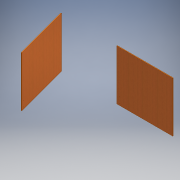
# Autodesk Inventor part: puerta
Saved by Autodesk Inventor 2016 (Build 200138000, 138)
## iProperties
Created: 2015-11-25
Part Number: puerta
Material: Generic
Document SubType Name: Modeling
Designer: Daniela
Density: 1 g/cm^3
Appearance: Glossy - Black
Author: Daniela
Autodesk Inventor part; units mm, degrees
ref_plane "YZ Plane" through (0, 0, 0) normal (1, 0, 0) x (0, 1, 0)
ref_plane "XZ Plane" through (0, 0, 0) normal (0, 1, 0) x (-1, 0, 0)
ref_plane "XY Plane" through (0, 0, 0) normal (0, 0, 1) x (1, 0, 0)
ref_plane "Plano de trabajo4" through (0, 0, 1220) normal (0, 0, 1) x (1, 0, 0)
sketch "Boceto8" plane through (0, 0, 1220) normal (0, 0, 1) x (1, 0, 0)
  line L0 (480, 0) -> (0, 0) projected
  line L1 (480, 0) -> (480, 10) projected
  line L2 (0, 10) -> (480, 10) projected
  line L3 (0, 0) -> (0, 10) projected
  line L4 (480, 10) -> (0, 10) projected
  line L5 (0, 10) -> (0, 300)
  line L6 (0, 300) -> (721.6667, 300)
  line L7 (721.6667, 300) -> (721.6667, 310)
  line L8 (721.6667, 310) -> (0, 310)
  line L9 (0, 310) -> (0, 300)
  point P0 (0, 0)
  dimension "d38" = 290
  dimension "d39" = 721.6667
  dimension "d40" = 10
  constraints: 10 end point, 2 parallel, 1 horizontal, 1 perpendicular, 1 vertical
  measures "d38" distance of L2.start L5.end
  measures "d39" distance of L8.end L7.end
  measures "d40" distance of L7.end L6.end
extrude "Extrusión8" add sketch "Boceto8" along normal blind 730 contours L9 L8 L7 L6
sketch "Boceto9" plane through (0, 300, 1220) normal (0, -1, 0) x (1, 0, 0)
  line L0 (0, 0) -> (721.6667, 0) construction
  line L1 (721.6667, 0) -> (721.6667, 730) construction
  line L2 (0, 730) -> (721.6667, 730) construction
  line L3 (0, 0) -> (0, 730) construction
  line L4 (0, 80) -> (721.6667, 80) construction
  line L5 (0, 0) -> (721.6667, 0) construction
  line L6 (36.0833, 0) -> (36.0833, 730) construction
  line L7 (0, 730) -> (721.6667, 730) construction
  circle A0 centre (36.0833, 30) radius 3
  circle A1 centre (36.0833, 130) radius 3
  point P0 (0, -1220)
  dimension "d43" = 36.0833
  dimension "d44" = 80
  dimension "d45" = 6
  dimension "d46" = 50
  constraints: 5 point on line, 4 end point, 2 centre point, 2 perpendicular, 1 symmetric about line, 1 other
  measures "d43" distance between parallel lines of L6 L3
  measures "d44" distance between parallel lines of L4 L0
  measures "d45" diameter of A0
  measures "d46" distance from line of L4 A0.centre
extrude "Extrusión9" cut sketch "Boceto9" against normal up to next
sketch "Boceto10" plane through (0, 0, 1950) normal (0, 0, 1) x (1, 0, 0)
  line L0 (721.6667, 310) -> (0, 310) projected
  line L1 (0, 310) -> (-721.6667, 310)
  line L2 (-721.6667, 310) -> (-534.8856, -387.0765)
  line L3 (-534.8856, -387.0765) -> (-544.5448, -389.6647)
  line L4 (-544.5448, -389.6647) -> (-731.3259, 307.4118)
  line L5 (-731.3259, 307.4118) -> (-721.6667, 310)
  point P0 (0, 0)
  dimension "d49" = 721.6667
  dimension "d50" = 721.6667
  dimension "angulo" = 75
  dimension "d52" = 10
  dimension "d53" = 721.6667
  constraints: 10 end point, 2 perpendicular, 1 horizontal
  measures "d49" distance of L0.end L1.end
  measures "d50" distance of L1.end L2.end
  measures "angulo" angle of L2 L1
  measures "d52" distance of L2.end L3.end
  measures "d53" distance of L3.end L4.end
extrude "Extrusión10" add sketch "Boceto10" against normal blind 730
sketch "Boceto11" plane through (-534.8856, -387.0765, 1950) normal (0.9659258, 0.258819, 0) x (0, 0, -1)
  line L0 (0, 721.6667) -> (0, 0) construction
  line L1 (0, 0) -> (730, 0) construction
  line L2 (730, 721.6667) -> (730, 0) construction
  line L3 (0, 721.6667) -> (730, 721.6667) construction
  line L4 (0, 721.6667) -> (0, 0) construction
  line L5 (0, 36.0833) -> (730, 36.0833) construction
  line L6 (0, 0) -> (730, 0) construction
  line L7 (650, 0) -> (650, 721.6667) construction
  line L8 (0, 721.6667) -> (730, 721.6667) construction
  circle A0 centre (700, 36.0833) radius 3
  circle A1 centre (600, 36.0833) radius 3
  point P0 (1950, 235.4486)
  dimension "d56" = 36.0833
  dimension "d57" = 80
  dimension "d58" = 6
  dimension "d59" = 50
  constraints: 5 point on line, 4 end point, 2 centre point, 2 perpendicular, 1 symmetric about line, 1 other
  measures "d56" distance between parallel lines of L1 L5
  measures "d57" distance between parallel lines of L2 L7
  measures "d58" diameter of A0
  measures "d59" distance from line of L7 A0.centre
extrude "Extrusión11" cut sketch "Boceto11" against normal up to next
equation "\"d39\" = ancho_m"
equation "\"d40\" = espesor"
equation "\"d43\" = 0.05 * ancho_m"
equation "\"d49\" = ancho_m"
equation "\"d50\" = ancho_m"
equation "\"d52\" = espesor"
equation "\"d53\" = ancho_m"
equation "\"d54\" = h_sup"
equation "\"d56\" = 0.05 * ancho_m"
equation "\"d60\" = h_sup"
equation "\"ancho_m\" = 721.666667"
equation "\"espesor\" = 10"
equation "\"h_sup\" = 730"
body "Solid1"
